Tesla Model Y Mason Jar Cupholder (Autodesk Fusion 360 design; units mm, degrees)
Autodesk Fusion 360 part; units mm, degrees
sketch "Frame" plane through (0, 0, 0) normal (0, 0, 1) x (1, 0, 0)
  line L0 (95, 79.5) -> (-95, 79.5)
  line L1 (-95, 79.5) -> (-95, -79.5)
  line L2 (-95, -79.5) -> (95, -79.5)
  line L3 (95, -79.5) -> (95, 79.5)
  line L4 (95, 79.5) -> (-95, -79.5) construction
  line L5 (-95, 79.5) -> (95, -79.5) construction
  line L6 (-90, -79.5) -> (90, -79.5)
  line L7 (90, -79.5) -> (90, 79.5)
  line L8 (90, 79.5) -> (-90, 79.5)
  line L9 (-90, 79.5) -> (-90, -79.5)
  line L10 (-90, -79.5) -> (90, 79.5) construction
  line L11 (90, -79.5) -> (-90, 79.5) construction
  line L12 (86, -75.5) -> (86, 75.5)
  line L13 (86, 75.5) -> (-86, 75.5)
  line L14 (-86, 75.5) -> (-86, -75.5)
  line L15 (-86, -75.5) -> (86, -75.5)
  dimension "d1" = 190
  dimension "d2" = 159
  dimension "d3" = 180
  dimension "d4" = -4
  constraint horizontal L0
  constraint perpendicular L0 L1
  constraint parallel L0 L2
  constraint parallel L1 L3
  constraint coincident L4 origin
  constraint coincident L5 origin
  constraint horizontal L6
  constraint perpendicular L6 L7
  constraint parallel L6 L8
  constraint parallel L7 L9
  constraint coincident L10 origin
  constraint coincident L11 origin
  constraint coincident L2 L6.start
  measures "d1" distance of L1.end L2.end
  measures "d2" distance of L0.end L1.end
  measures "d3" distance of L7 L9
extrude "Extrude1" add sketch "Frame" against normal blind 6 contours L0 L2 L6 L7 L8 L9 makes body 1
extrude "Extrude2" add sketch "Frame" along normal blind 4 bodies 1
sketch "Jar Hole" plane through (0, 0, 4) normal (0, 0, -1) x (1, 0, 0)
  line L0 (-86, 75.5) -> (86, 75.5)
  line L1 (86, 75.5) -> (86, -75.5)
  line L2 (86, -75.5) -> (-86, -75.5)
  line L3 (-90, 79.5) -> (-90, -79.5)
  line L4 (-90, -79.5) -> (90, -79.5)
  line L5 (90, -79.5) -> (90, 79.5)
  line L6 (90, 79.5) -> (-90, 79.5)
  line L7 (60, 70.5) -> (60, -49.5)
  line L8 (60, -49.5) -> (-60, -49.5)
  line L9 (86, 75.5) -> (46, 75.5)
  line L10 (86, 21.5) -> (86, 75.5)
  line L11 (86, -56.5) -> (86, 9.1429)
  line L12 (60, 70.5) -> (-60, 70.5)
  line L13 (-60, 70.5) -> (-60, -49.5)
  line L14 (-86, 75.5) -> (-86, -75.5)
  line L15 (86, 75.5) -> (-86, 75.5)
  line L16 (64, 74.5) -> (64, -53.5)
  line L17 (64, -53.5) -> (-64, -53.5)
  line L18 (-64, 74.5) -> (-64, -53.5)
  line L19 (64, 74.5) -> (-64, 74.5)
  line L20 (86, 75.5) -> (-86, 75.5)
  line L21 (-86, 75.5) -> (-86, -75.5)
  line L22 (-86, -75.5) -> (86, -75.5)
  line L23 (86, -75.5) -> (86, 75.5)
  line L24 (95, -79.5) -> (-95, -79.5)
  line L25 (-95, -79.5) -> (-95, 79.5)
  line L26 (-95, 79.5) -> (95, 79.5)
  line L27 (95, 79.5) -> (95, -79.5)
  dimension "d11" = 40
  dimension "d12" = 54
  dimension "d25" = 120
  dimension "d26" = 120
  dimension "d35" = -4
  dimension "d36" = 22
  dimension "d37" = 1
  constraint vertical L7
  constraint horizontal L8
  constraint horizontal L9
  constraint vertical L10
  constraint coincident L0.end L1.start
  constraint vertical L11
  constraint coincident L1 L11.end
  constraint perpendicular L7 L12
  constraint perpendicular L8 L13
  measures "d11" distance of L0.end L9.end
  measures "d12" distance of L0.end L10.start
  measures "d25" distance of L7.start L12.end
  measures "d26" distance of L8 L12
  measures "d36" distance of L14 L18
  measures "d37" vertical distance of L0.start L18.start
extrude "Extrude3" add sketch "Jar Hole" along normal blind 10 contours L0 L1 L2 L9 L10 L11 L14 L15 L20 L21 L22 L23 | L16 L17 L18 L19 bodies 1
extrude "Extrude8" add sketch "Jar Hole" along normal blind 88.9 contours L16 L17 L18 L19 bodies 1
sketch "Sketch Bottom Lid" plane through (0, 0, -84.9) normal (0, 0, -1) x (1, 0, 0)
  line L0 (-60, 70.5) -> (60, 70.5)
  line L1 (60, 70.5) -> (60, -49.5)
  line L2 (60, -49.5) -> (-60, -49.5)
  line L3 (-60, -49.5) -> (-60, 70.5)
  line L4 (64, -53.5) -> (64, 74.5)
  line L5 (64, 74.5) -> (-64, 74.5)
  line L6 (-64, 74.5) -> (-64, -53.5)
  line L7 (-64, -53.5) -> (64, -53.5)
  line L8 (64, 74.5) -> (64, -53.5)
  line L9 (64, -53.5) -> (-64, -53.5)
  line L10 (-64, 74.5) -> (-64, -53.5)
  line L11 (64, 74.5) -> (-64, 74.5)
  line L12 (-66, 76.5) -> (-66, -55.5)
  line L13 (66, -55.5) -> (-66, -55.5)
  line L14 (66, 76.5) -> (66, -55.5)
  line L15 (66, 76.5) -> (-66, 76.5)
  dimension "d44" = -2
extrude "Extrude9" add sketch "Sketch Bottom Lid" against normal blind 2 separate body contours L12 L13 L14 L15 makes body 2
extrude "Extrude10" add sketch "Sketch Bottom Lid" along normal blind 3 contours L0 L1 L2 L3 | L4 L5 L6 L7 L8 L9 L10 L11 | L12 L13 L14 L15 bodies 2
fillet "Fillet2" radius 5 4 edges at (-60, 49.5, -40.45) (60, -70.5, -40.45) (-60, -70.5, -40.45) (60, 49.5, -40.45) on bodies 1
chamfer "Chamfer1" distance 2 angle 45 8 edges at (60, -10.5, 4) (58.5355, 48.0355, 4) (0, 49.5, 4) (-58.5355, 48.0355, 4) (-60, -10.5, 4) (-58.5355, -69.0355, 4) (0, -70.5, 4) (58.5355, -69.0355, 4) on bodies 1
chamfer "Chamfer2" distance 3 angle 45 4 edges at (0, -74.5, -6) (-64, -10.5, -6) (0, 53.5, -6) (64, -10.5, -6) on bodies 1
named bodies: "Base", "Bottom"
